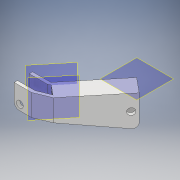
# Autodesk Inventor part: Thumb1
Saved by Autodesk Inventor 2018 (Build 220112000, 112)
## iProperties
Created: 2018-02-21
Part Number: Thumb1
Material: Plastique ABS
Document SubType Name: Modeling
Designer: Thomas
Density: 1.06 g/cm^3
Appearance: Lisse - Blanc
Author: Thomas
Autodesk Inventor part; units mm, degrees
ref_plane "YZ Plane" through (0, 0, 0) normal (1, 0, 0) x (0, 1, 0)
ref_plane "XZ Plane" through (0, 0, 0) normal (0, 1, 0) x (-1, 0, 0)
ref_plane "XY Plane" through (0, 0, 0) normal (0, 0, 1) x (1, 0, 0)
sketch "Esquisse1" plane through (0, 0, 0) normal (0, 0, 1) x (1, 0, 0)
  line L0 (0, 0) -> (0, 2)
  line L1 (0, 2) -> (10.4, 2)
  line L2 (0, 0) -> (10.4, 0)
  line L3 (10.4, 0) -> (19.648, 3.8307)
  line L4 (0, 9) -> (10.7082, 9)
  line L5 (0, 11) -> (0, 9)
  line L6 (0, 11) -> (10.9257, 11)
  line L7 (10.4, 2) -> (18.103, 5.1006)
  line L8 (18.103, 5.1006) -> (19.648, 3.8307)
  line L9 (10.9257, 11) -> (19.648, 3.8307) construction
  line L10 (10.9257, 11) -> (12.2416, 9.9184) construction
  line L11 (10.9257, 11) -> (12.4707, 9.73)
  line L12 (10.7082, 9) -> (12.4707, 9.73)
  dimension "d0" = 2
  dimension "d1" = 10.4
  dimension "d2" = 10.4
  dimension "d3" = 157.5
  dimension "d5" = 10.01
  dimension "d8" = 7
  dimension "d26" = 2
  dimension "d32" = 2
  dimension "d33" = 2
  dimension "d34" = 157.5
  constraints: 26 end point, 3 horizontal, 1 perpendicular, 1 point on line, 1 vertical
  measures "d0" distance of L0.start L0.end
  measures "d1" distance of L0.end L1.end
  measures "d2" distance of L0.start L2.end
  measures "d3" angle of L3 L2
  measures "d5" distance of L2.end L3.end
  measures "d8" vertical distance of L1.end L4.end
  measures "d26" distance of L5.start L4.start
  measures "d32" distance of L7.end L3.end
  measures "d33" distance of L6.end L11.end
  measures "d34" angle of L12 L4
extrude "Extrusion1" add sketch "Esquisse1" along normal blind 13
sketch "Esquisse4" plane through (0, 0, 0) normal (0, -1, 0) x (1, 0, 0)
  circle A0 centre (3.39, 3.39) radius 2
  line L0 (0, 13) -> (10.4, 13) projected
  line L1 (0, 0) -> (0, 13) projected
  line L2 (10.4, 0) -> (0, 0) projected
  point P0 (3, 13)
  point P1 (0, 10)
  dimension "d35" = 4
  dimension "d37" = 3.39
  dimension "d50" = 3.39
  constraints: 1 centre point
  measures "d35" diameter of A0
  measures "d37" distance from line of L1 A0.centre
  measures "d50" distance from line of L2 A0.centre
extrude "Extrusion3" cut sketch "Esquisse4" against normal blind 13
ref_plane "Plan de construction3" through (19.648, 3.8307, 13) normal (-0.7725294, 0.634979, 0) x (-0.634979, -0.7725294, 0)
sketch "Esquisse5" plane through (19.648, 3.8307, 13) normal (-0.7725294, 0.634979, 0) x (-0.634979, -0.7725294, 0)
  line L0 (0, 0) -> (6.9376, 0) projected
  line L1 (0, -13) -> (6.9376, -13) projected
  line L2 (0, 0) -> (0, -13)
  line L3 (0, -13) -> (-32.924, -18.2914)
  line L4 (-36.4, -15.3294) -> (-36.4, 0)
  line L5 (-36.4, 0) -> (0, 0)
  arc A0 (-36.4, -15.3294) -> (-32.924, -18.2914) centre (-33.4, -15.3294) ccw
  point P0 (15.4354, -13)
  point P1 (5.0326, 0)
  point P2 (-36.4, -18.85)
  dimension "d40" = 36.4
  dimension "d41" = 18.85
  dimension "d42" = 3
  constraints: 8 end point, 2 point on circle, 2 point on line, 2 tangent, 1 centre point, 1 parallel, 1 perpendicular, 1 vertical
  measures "d40" distance of L4.end L0.start
  measures "d41" distance of point (-36.4, -18.85) L4.end
  measures "d42" radius of A0
extrude "Extrusion4" add sketch "Esquisse5" along normal blind 2
ref_plane "Plan de construction4" through (12.4707, 9.73, 13) normal (-0.7725294, 0.634979, 0) x (-0.634979, -0.7725294, 0)
sketch "Esquisse6" plane through (12.4707, 9.73, 13) normal (-0.7725294, 0.634979, 0) x (-0.634979, -0.7725294, 0)
  line L0 (0, -13) -> (0, 0) projected
  line L1 (0, -13) -> (0, 0) projected
  line L2 (0, -13) -> (0, 0)
  line L3 (0, 0) -> (-36.4, 0)
  line L4 (-36.4, 0) -> (-36.4, -15.3294) projected
  line L5 (-36.4, 0) -> (-36.4, -15.3294)
  line L6 (-32.924, -18.2914) -> (0, -13)
  arc A0 (-36.4, -15.3294) -> (-32.924, -18.2914) centre (-33.4, -15.3294) ccw
  point P0 (15.4354, -13)
  point P1 (-36.4, -18.85)
  dimension "d45" = 36.4
  dimension "d46" = 18.85
  dimension "d47" = 3
  constraints: 8 end point, 2 collinear, 2 point on circle, 2 point on line, 2 tangent, 1 centre point, 1 perpendicular
  measures "d45" distance of L0.end L3.end
  measures "d46" distance of L3.end point (-36.4, -18.85)
  measures "d47" radius of A0
extrude "Extrusion5" add sketch "Esquisse6" along normal blind 2
fillet "Congé4" radius 3 2 edges at (0, 1, 0) (0, 10, 0)
ref_plane "Plan de construction6" through (34.8114, 38.4851, 13) normal (0, 0, -1) x (-1, 0, 0)
sketch "Esquisse8" plane through (34.8114, 38.4851, 13) normal (0, 0, -1) x (-1, 0, 0)
  line L0 (1.4347, -3.3203) -> (-0.7725, -0.635) projected
  line L1 (24.1032, -29.4851) -> (22.3407, -28.755) projected
  line L2 (-0.7725, -0.635) -> (22.3407, -28.755)
  line L3 (16.7085, -33.3845) -> (-6.4048, -5.2644) projected
  line L4 (22.3407, -28.755) -> (16.7085, -33.3845)
  line L5 (16.7085, -33.3845) -> (-6.4048, -5.2644)
  line L6 (-6.4048, -5.2644) -> (-0.7725, -0.635)
  point P0 (34.8114, -38.4851)
  constraints: 8 end point, 2 perpendicular, 1 collinear
extrude "Extrusion6" add sketch "Esquisse8" along normal blind 2
sketch "Esquisse9" plane through (19.648, 3.8307, 13) normal (0.7725294, -0.634979, 0) x (0, 0, -1)
  circle A0 centre (9.425, 33.01) radius 2
  line L0 (18.2914, 32.924) -> (13, 0) construction
  line L1 (17.0751, 25.3561) -> (18.85, 36.4) construction
  line L2 (18.85, 36.4) -> (0, 36.4) construction
  line L3 (0, 36.4) -> (0, 0) construction
  point P0 (13, -15.4354)
  dimension "d54" = 3.39
  dimension "d55" = 9.425
  dimension "d56" = 4
  constraints: 4 end point, 1 centre point, 1 collinear, 1 horizontal, 1 point on line
  measures "d54" distance from line of L2 A0.centre
  measures "d55" distance from line of L3 A0.centre
  measures "d56" diameter of A0
extrude "Extrusion7" cut sketch "Esquisse9" against normal blind 13
